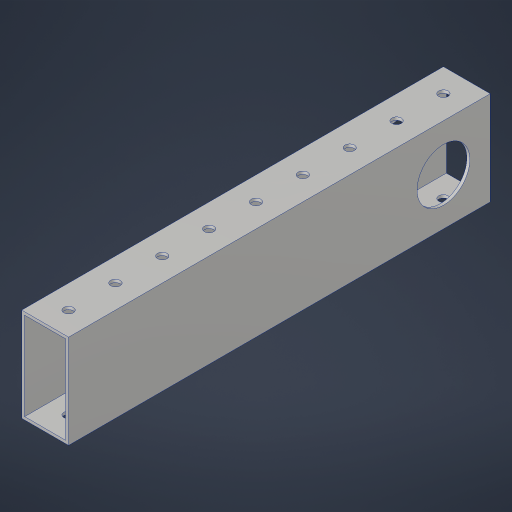
# Autodesk Inventor part: CL3-001
Saved by Autodesk Inventor 2023.4 (Build 274418000, 418)
## iProperties
RuleStatus: InUse
Created: 2025-01-28
Part Number: CL3-001
Material: Aluminum 6061
Document SubType Name: Modeling
Designer: slick
Mass: 304.185 g
Surface Area: 718.547 cm^2
Volume: 112.661 cm^3
Density: 2.7 g/cm^3
Appearance: Aluminum - Flat
AfterDocNew0: SHOW
AfterDocOpen0: SHOW
Author: slick
Autodesk Inventor part; units mm, degrees
ref_plane "YZ Plane" through (0, 0, 0) normal (1, 0, 0) x (0, 1, 0)
ref_plane "XZ Plane" through (0, 0, 0) normal (0, 1, 0) x (-1, 0, 0)
ref_plane "XY Plane" through (0, 0, 0) normal (0, 0, 1) x (1, 0, 0)
sketch "Sketch1" plane through (0, 0, 0) normal (0, 0, 1) x (1, 0, 0)
  line L0 (-12.7, -25.4) -> (12.7, -25.4)
  line L1 (12.7, -25.4) -> (12.7, 25.4)
  line L2 (12.7, 25.4) -> (-12.7, 25.4)
  line L3 (-12.7, 25.4) -> (-12.7, -25.4)
  line L4 (-12.7, -25.4) -> (12.7, 25.4) construction
  line L5 (12.7, -25.4) -> (-12.7, 25.4) construction
  line L6 (-11.1125, 23.8125) -> (11.1125, 23.8125)
  line L7 (11.1125, 23.8125) -> (11.1125, -23.8125)
  line L8 (11.1125, -23.8125) -> (-11.1125, -23.8125)
  line L9 (-11.1125, -23.8125) -> (-11.1125, 23.8125)
  point P0 (0, 0)
  dimension "width" = 25.4
  dimension "height" = 50.8
  dimension "thickness" = 1.5875
  constraints: 20 end point, 4 parallel, 2 midpoint, 2 perpendicular, 1 horizontal, 3 other
  measures "width" distance of L2.end L1.end
  measures "height" distance of L1.end L0.end
  measures "thickness" distance between parallel lines of L2 L6
extrude "Extrusion1" add sketch "Sketch1" along normal mid plane 228.6
sketch "Sketch3" plane through (-12.7, -25.4, -114.3) normal (-1, 0, 0) x (0, 0, 1)
  circle A0 centre (25.4, 25.4) radius 14.2875
  line L0 (0, 0) -> (0, 50.8) projected
  point P0 (114.3, 25.4)
  dimension "d8" = 28.575
  dimension "d9" = 25.4
  constraints: 1 centre point, 1 horizontal alignment
  measures "d8" diameter of A0
  measures "d9" distance from line of L0 A0.centre
extrude "Extrusion3" cut sketch "Sketch3" against normal through all
sketch "Sketch4" plane through (-12.7, 25.4, 114.3) normal (0, 1, 0) x (1, 0, 0)
  line L0 (0, 228.6) -> (0, 0) projected
  line L1 (25.4, 0) -> (0, 0) projected
  line L2 (25.4, 228.6) -> (25.4, 0) projected
  line L3 (0, 228.6) -> (25.4, 228.6) construction
  line L4 (0, 228.6) -> (0, 0) construction
  line L5 (25.4, 228.6) -> (25.4, 0) construction
  line L6 (0, 0) -> (25.4, 0) construction
  line L7 (25.4, 0) -> (0, 25.4)
  line L8 (0, 25.4) -> (0, 0)
  line L9 (0, 0) -> (25.4, 0)
  point P0 (12.7, 114.3)
  point P1 (0, 25.4)
  dimension "d17" = 45
  constraints: 6 end point, 2 collinear, 1 point on line
  measures "d17" angle of L1 L7
extrude "Extrusion4" [suppressed]
sketch "Sketch5" plane through (-12.7, 25.4, -114.3) normal (0, 1, 0) x (1, 0, 0)
  line L0 (0, 0) -> (25.4, 0) construction
  line L1 (25.4, 0) -> (25.4, -228.6) construction
  line L2 (0, -228.6) -> (0, 0) construction
  line L3 (25.4, -228.6) -> (0, -228.6) projected
  point P0 (12.7, -114.3)
  point P1 (12.7, -12.7)
  point P2 (12.7, 0)
  dimension "d18" = 12.7
  constraints: 1 midpoint, 1 vertical alignment
  measures "d18" distance from line of L0 point (12.7, -12.7)
hole "Hole1" at (0, 25.4, -101.6) direction (0, -1, 0) diameter 5.1054 end through all clearance for "Flat Head Machine Screw (82)" size "#10" standard "Ansi Unified Screw Threads"
pattern_linear "Rectangular Pattern1" count 9 spacing 25.4 along (0, 0, 1) of "Hole1"
sketch "Sketch6" plane through (-12.7, 25.4, 114.3) normal (0, 1, 0) x (1, 0, 0)
  circle A0 centre (12.7, 38.1) radius 2.5527 construction
  circle A1 centre (12.7, 63.5) radius 2.5527 construction
  circle A2 centre (12.7, 88.9) radius 2.5527 construction
  circle A3 centre (12.7, 114.3) radius 2.5527 construction
  circle A4 centre (12.7, 139.7) radius 2.5527 construction
  circle A5 centre (12.7, 165.1) radius 2.5527 construction
  circle A6 centre (12.7, 190.5) radius 2.5527 construction
  circle A7 centre (12.7, 215.9) radius 2.5527 construction
  line L0 (0, 228.6) -> (25.4, 228.6) construction
  line L1 (25.4, 228.6) -> (25.4, 0) construction
  line L2 (25.4, 0) -> (0, 0) construction
  line L3 (0, 0) -> (0, 228.6) construction
  line L4 (25.4, 0) -> (25.4, 25.4)
  line L5 (25.4, 25.4) -> (0, 0)
  line L6 (0, 0) -> (25.4, 0)
  circle A8 centre (12.7, 12.7) radius 2.5527 projected
  dimension "d29" = 45
  constraints: 6 end point, 1 vertical
  measures "d29" angle of L2 L5
extrude "Extrusion5" [suppressed]
body "Solid1"
